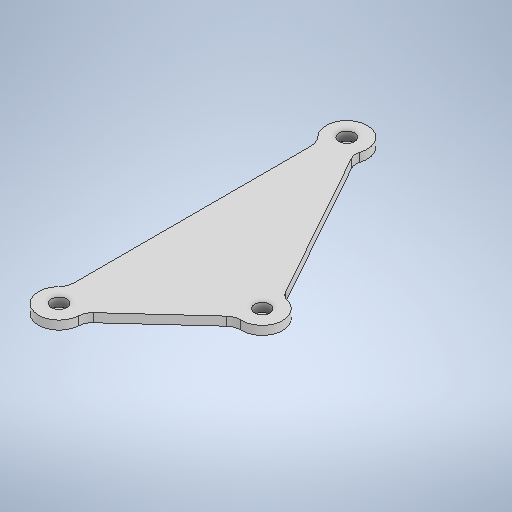
# Autodesk Inventor part: A2P2
Saved by Autodesk Inventor 2025.2 (Build 292293000, 293)
## iProperties
Created: 2025-05-22
Part Number: A2P2
Material: Generic
Document SubType Name: Sheet Metal
Designer: Admin
Density: 1 g/cm^3
Sheet Metal Rule: Default
Appearance: Default
Author: Admin
Autodesk Inventor part; units mm, degrees
ref_plane "YZ Plane" through (0, 0, 0) normal (1, 0, 0) x (0, 1, 0)
ref_plane "XZ Plane" through (0, 0, 0) normal (0, 1, 0) x (-1, 0, 0)
ref_plane "XY Plane" through (0, 0, 0) normal (0, 0, 1) x (1, 0, 0)
sketch "Sketch1" plane through (0, 0, 0) normal (0, 1, 0) x (-1, 0, 0)
  circle A0 centre (0, 0) radius 4
  line L0 (2, -5) -> (2, -51.029)
  line L1 (-2, -7.543) -> (-2, -44.0823)
  circle A1 centre (0, -56.029) radius 4
  circle A2 centre (-20.6662, -18.892) radius 4
  line L2 (-4.2179, -6.5655) -> (-15.9345, -17.2762)
  line L3 (-4.9298, -1.7969) -> (-18.4353, -14.1429)
  line L4 (-16.6903, -21.9238) -> (-4.0616, -44.6173)
  line L5 (-20.1855, -23.8688) -> (-3.976, -52.9972)
  arc A3 (2.8966, -2.7586) -> (2, -5) centre (5.25, -5) ccw
  arc A4 (2, -51.029) -> (2.8966, -53.2704) centre (5.25, -51.029) ccw
  arc A5 (-4.9298, -1.7969) -> (-3.9954, 0.1924) centre (-6.875, 0.331) ccw
  arc A6 (-20.5001, -14.8954) -> (-18.4353, -14.1429) centre (-20.3803, -12.0152) ccw
  line L6 (0, 0) -> (-20.6662, -18.892) construction
  line L7 (-20.6662, -18.892) -> (0, -56.029) construction
  arc A7 (-15.9345, -17.2762) -> (-16.6663, -18.9207) centre (-14.4164, -18.9369) ccw
  arc A8 (-16.8633, -20.1321) -> (-16.6903, -21.9238) centre (-14.7242, -20.8297) ccw
  arc A9 (-2, -7.543) -> (-4.2179, -6.5655) centre (-3.3243, -7.543) ccw
  arc A10 (-4.0616, -44.6173) -> (-2, -44.0823) centre (-3.1002, -44.0823) ccw
  arc A11 (-20.1855, -23.8688) -> (-21.6168, -22.7774) centre (-22.1516, -24.9629) ccw
  arc A12 (-3.8029, -54.7889) -> (-3.976, -52.9972) centre (-5.942, -54.0913) ccw
  point P0 (-21.4801, -12.8095)
  dimension "d0" = 8
  dimension "d1" = 8
  dimension "d2" = 8
  dimension "d4" = 42.5
  dimension "d5" = 28
  dimension "d6" = 2
  dimension "d7" = 2
  dimension "d8" = 5
  dimension "d10" = 5
  dimension "d11" = 0
  dimension "d12" = 5.2471
  dimension "d14" = 5.247
  dimension "d15" = 2
  dimension "d16" = 2
  dimension "d17" = 2
  dimension "d18" = 2
  dimension "d19" = 4
  dimension "d20" = 5
  dimension "d21" = 5
  dimension "d22" = 5
  dimension "d23" = 1.1002
  dimension "d24" = 1.3243
  dimension "d38" = 56.029
  constraints: 28 point on circle, 20 tangent, 16 end point, 13 centre point, 4 parallel, 2 vertical, 1 coincident
  measures "d0" diameter of A0
  measures "d1" diameter of A1
  measures "d2" diameter of A2
  measures "d4" distance of L6.end L7.end
  measures "d5" distance of point (0, 0) L6.end
  measures "d6" horizontal distance of point (0, 0) L0.start
  measures "d7" horizontal distance of point (0, 0) L1.start
  measures "d8" vertical distance of point (0, 0) L0.start
  measures "d10" vertical distance of L7.end L0.end
  measures "d11" horizontal distance of L7.end point (0, 0)
  measures "d12" distance of L3.start point (0, 0)
  measures "d14" distance of L6.end L3.end
  measures "d15" distance from line of L6 L3.start
  measures "d16" distance from line of L6 L2.end
  measures "d17" distance from line of L7 L4.end
  measures "d18" distance from line of L7 L5.end
  measures "d19" distance of L4.start L5.start
  measures "d20" distance of L5.end L7.end
  measures "d21" distance of L6.end L4.start
  measures "d22" distance of L6.end L2.end
  measures "d23" distance from line of L4 A10.centre
  measures "d24" radius of A9
  measures "d38" distance of point (0, 0) L7.end
extrude "Extrusion1" add sketch "Sketch1" along normal blind 4 contours A0 | A2 | A1
extrude "Extrusion2" add sketch "Sketch1" along normal blind 1.7 contours A0 A3 L0 A4 A1 A12 L5 A11 A2 A8 L4 A10 L1 A9 L2 A7 A6 L3 A5 | A7 L2 A9 L1 A10 L4 A8 A2
sketch "Sketch2" plane through (0, 4, 0) normal (0, 1, 0) x (1, 0, 0)
  circle A0 centre (0, 0) radius 4 projected
  circle A1 centre (0, 0) radius 1.5
  circle A2 centre (20.6662, 18.892) radius 4 projected
  circle A3 centre (20.6662, 18.892) radius 1.5
  circle A4 centre (0, 56.029) radius 1.5
  circle A5 centre (0, 56.029) radius 4 projected
  dimension "d29" = 3
  dimension "d30" = 3
  dimension "d31" = 3
  dimension "d36" = 0
  constraints: 3 centre point, 2 coincident
  measures "d29" diameter of A1
  measures "d30" diameter of A4
  measures "d31" diameter of A3
  measures "d36" distance of A5.centre A4.centre
extrude "Extrusion3" cut sketch "Sketch2" against normal blind 4 contours A1 | A3 | A4
sketch "Sketch3" plane through (-2, 0, -51.029) normal (-1, 0, 0) x (0, 0, 1)
  line L0 (60.4555, 1.7) -> (-13.4083, 1.7)
  line L1 (-13.4083, 1.7) -> (-13.4083, 27.1644)
  line L2 (-13.4083, 27.1644) -> (60.4555, 27.1644)
  line L3 (60.4555, 27.1644) -> (60.4555, 1.7)
  point P0 (51.029, 0)
  constraints: 8 end point, 2 parallel, 1 horizontal, 1 perpendicular
extrude "Extrusion4" cut sketch "Sketch3" along normal mid plane 100
equation "\"BendRadius\" = Thickness"
equation "\"BendReliefWidth\" = Thickness"
equation "\"BendReliefDepth\" = 0.5 * Thickness"
equation "\"CornerReliefSize\" = 4 * Thickness"
equation "\"MinimumRemnant\" = 2 * Thickness"
equation "\"TransitionRadius\" = BendRadius"
equation "\"JacobiRadiusSize\" = BendRadius"
equation "\"GapSize\" = Thickness"
equation "\"Thickness\" = 3.048"
body "Solid1"
